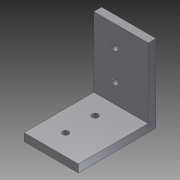
# Autodesk Inventor part: Corner
Saved by Autodesk Inventor 2014 (Build 180170000, 170)
## iProperties
Created: 2012-10-17
Material: Generic
Document SubType Name: Modeling
Density: 1 g/cm^3
Appearance: Default
Autodesk Inventor part; units mm, degrees
ref_plane "YZ Plane" through (0, 0, 0) normal (1, 0, 0) x (0, 1, 0)
ref_plane "XZ Plane" through (0, 0, 0) normal (0, 1, 0) x (-1, 0, 0)
ref_plane "XY Plane" through (0, 0, 0) normal (0, 0, 1) x (1, 0, 0)
sketch "Sketch1" plane through (0, 0, 0) normal (0, 0, 1) x (1, 0, 0)
  line L0 (0, 5) -> (45, 5)
  line L1 (45, 5) -> (45, 50)
  line L2 (45, 50) -> (50, 50)
  line L3 (50, 50) -> (50, 0)
  line L4 (50, 0) -> (0, 0)
  line L5 (0, 0) -> (0, 5)
  dimension "d0" = 50
  dimension "d1" = 50
  dimension "d2" = 5
  dimension "d3" = 5
  constraints: 12 end point, 5 perpendicular, 1 coincident, 1 horizontal
  measures "d0" distance of L3.end L4.end
  measures "d1" distance of L2.end L3.end
  measures "d2" distance of L1.end L2.end
  measures "d3" distance of L4.end L0.start
extrude "Extrusion1" add sketch "Sketch1" along normal mid plane 35
sketch "Sketch2" plane through (0, 5, 17.5) normal (0, 1, 0) x (1, 0, 0)
  line L0 (45, 35) -> (0, 35) projected
  line L1 (0, 35) -> (0, 0) projected
  circle A0 centre (13.2, 21.5) radius 2
  circle A1 centre (32.3, 21.5) radius 2
  point P0 (0, 17.5)
  dimension "d6" = 4
  dimension "d7" = 13.2
  dimension "d8" = 19.1
  dimension "d9" = 13.5
  constraints: 2 centre point, 1 equal radius, 1 horizontal alignment
  measures "d6" diameter of A0
  measures "d7" distance from line of A0.centre L1
  measures "d8" distance of A1.centre A0.centre
  measures "d9" distance from line of L0 A0.centre
extrude "Extrusion2" cut sketch "Sketch2" against normal through all
sketch "Sketch3" plane through (45, 5, 17.5) normal (-1, 0, 0) x (0, 0, 1)
  line L0 (0, 45) -> (-35, 45) projected
  line L1 (-35, 45) -> (-35, 0) projected
  circle A0 centre (-21.5, 31.8) radius 2
  circle A1 centre (-21.5, 12.7) radius 2
  point P0 (-17.5, -5)
  dimension "d12" = 13.2
  dimension "d13" = 19.1
  dimension "d14" = 13.5
  dimension "d15" = 4
  constraints: 2 centre point, 1 equal radius, 1 vertical alignment
  measures "d12" distance from line of L0 A0.centre
  measures "d13" distance of A0.centre A1.centre
  measures "d14" distance from line of L1 A0.centre
  measures "d15" diameter of A0
extrude "Extrusion3" cut sketch "Sketch3" against normal through all
body "Solid1"
